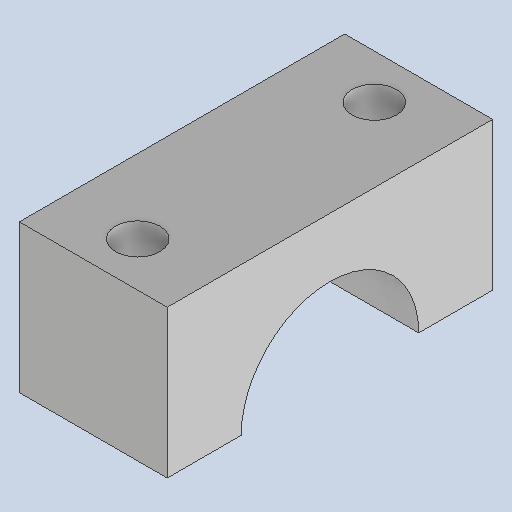
# Autodesk Inventor part: 145 part
Saved by Autodesk Inventor 2025.1 (Build 291241000, 241)
## iProperties
Created: 2024-08-01
Part Number: 145 part
Material: Generic
Document SubType Name: Modeling
Designer: ffogue
Density: 1 g/cm^3
Appearance: Default
Author: ffogue
Autodesk Inventor part; units mm, degrees
ref_plane "YZ Plane" through (0, 0, 0) normal (1, 0, 0) x (0, 1, 0)
ref_plane "XZ Plane" through (0, 0, 0) normal (0, 1, 0) x (-1, 0, 0)
ref_plane "XY Plane" through (0, 0, 0) normal (0, 0, 1) x (1, 0, 0)
sketch "Sketch1" plane through (0, 0, 0) normal (0, 0, 1) x (1, 0, 0)
  circle A0 centre (-5, -3) radius 1.5 projected
  line L0 (-10, -5) -> (0, -5) projected
  line L1 (0, 0) -> (0, -5) projected
  line L2 (-10, 0) -> (0, 0) projected
  line L3 (-10, 0) -> (-10, -5) projected
  circle A1 centre (-5, -3) radius 1.5 projected
  circle A2 centre (-5, -19) radius 1.5 projected
  line L4 (0, -17) -> (-10, -17) projected
  line L5 (-10, -17) -> (-10, -22) projected
  line L6 (0, -22) -> (-10, -22) projected
  line L7 (0, -17) -> (0, -22) projected
  circle A3 centre (-5, -19) radius 1.5 projected
  line L8 (-10, -17) -> (-10, -5) projected
  line L9 (0, -5) -> (0, -17) projected
extrude "Extrusion1" add sketch "Sketch1" along normal blind 10
sketch "Sketch2" plane through (-10, -22, 0) normal (-1, 0, 0) x (0, 0, 1)
  line L0 (0, 22) -> (0, 0) projected
  arc A0 (0, 5) -> (0, 17) centre (0, 11) ccw
  dimension "d2" = 12
  constraints: 2 point on circle, 2 point on line, 1 centre point, 1 midpoint
  measures "d2" diameter of A0
extrude "Extrusion2" cut sketch "Sketch2" against normal up to surface (10 mm away)
body "Solid1"
